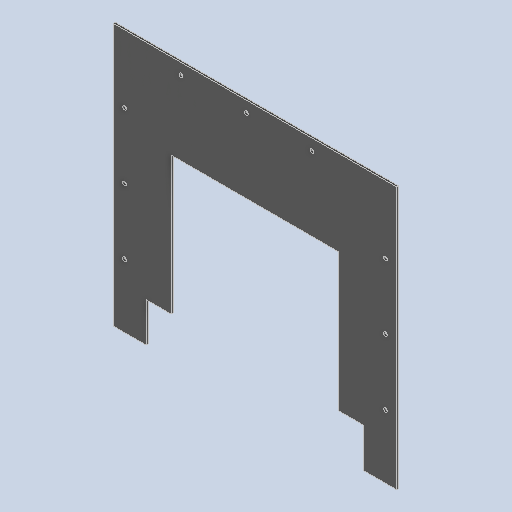
# Autodesk Inventor part: HCMUTE-CDT23-KXL_A03
Saved by Autodesk Inventor 2023 (Build 270158000, 158)
## iProperties
Created: 2023-11-20
Part Number: HCMUTE-CDT23-KXL_A03
Material: PMMA Plastic
Document SubType Name: Modeling
Designer: havie
Density: 1.188 g/cm^3
Appearance: Dark Gray
Author: havie
Autodesk Inventor part; units mm, degrees
ref_plane "YZ Plane" through (0, 0, 0) normal (1, 0, 0) x (0, 1, 0)
ref_plane "XZ Plane" through (0, 0, 0) normal (0, 1, 0) x (-1, 0, 0)
ref_plane "XY Plane" through (0, 0, 0) normal (0, 0, 1) x (1, 0, 0)
sketch "Sketch1" plane through (0, 0, 0) normal (1, 0, 0) x (0, 1, 0)
  line L0 (-216, 200) -> (216, 200)
  line L1 (216, 200) -> (216, -200)
  line L2 (216, -200) -> (-216, -200)
  line L3 (-216, -200) -> (-216, 200)
  line L4 (-216, 200) -> (216, -200) construction
  line L5 (216, 200) -> (-216, -200) construction
  point P0 (0, 0)
  dimension "d0" = 400
  dimension "d1" = 432
  constraints: 12 end point, 2 midpoint, 2 parallel, 1 horizontal, 1 perpendicular
  measures "d0" distance of L0.end L1.end
  measures "d1" distance of L1.end L2.end
extrude "Extrusion1" add sketch "Sketch1" along normal mid plane 3
sketch "Sketch2" plane through (1.5, 0, 0) normal (1, 0, 0) x (0, 0, -1)
  line L0 (200, 216) -> (-200, 216) projected
  line L1 (-200, -216) -> (200, -216) projected
  line L2 (200, -216) -> (200, 216) projected
  line L3 (200, 166) -> (140, 166)
  line L4 (140, 166) -> (140, 128)
  line L5 (140, 128) -> (-70, 128)
  line L6 (-70, 128) -> (-70, -128)
  line L7 (-70, -128) -> (140, -128)
  line L8 (140, -128) -> (140, -166)
  line L9 (140, -166) -> (200, -166)
  point P0 (0, 0)
  dimension "d6" = 50
  dimension "d7" = 50
  dimension "d8" = 60
  dimension "d9" = 38
  dimension "d10" = 270
  constraints: 14 end point, 5 perpendicular, 2 equal length, 2 point on line, 1 horizontal, 1 vertical
  measures "d6" distance between parallel lines of L0 L3
  measures "d7" distance between parallel lines of L1 L9
  measures "d8" distance of L3.start L3.end
  measures "d9" distance of L3.end L4.end
  measures "d10" distance between parallel lines of L2 L6
extrude "Extrusion2" cut sketch "Sketch2" against normal blind 3
sketch "Sketch3" plane through (-1.5, 0, 0) normal (-1, 0, 0) x (0, 0, 1)
  circle A0 centre (97, -199) radius 3
  circle A1 centre (-3, -199) radius 3
  circle A2 centre (-103, -199) radius 3
  line L0 (-200, -216) -> (200, -216) projected
  line L1 (200, -216) -> (200, 216) projected
  point P0 (0, 0)
  dimension "d15" = 6
  dimension "d16" = 6
  dimension "d17" = 6
  dimension "d18" = 17
  dimension "d19" = 103
  dimension "d20" = 100
  dimension "d21" = 100
  constraints: 3 centre point, 2 horizontal alignment
  measures "d15" diameter of A2
  measures "d16" diameter of A1
  measures "d17" diameter of A0
  measures "d18" distance from line of L0 A0.centre
  measures "d19" distance from line of L1 A0.centre
  measures "d20" distance of A1.centre A0.centre
  measures "d21" distance of A2.centre A1.centre
extrude "Extrusion3" cut sketch "Sketch3" against normal blind 3
mirror "Mirror1" about plane through (0, 0, 0) normal (0, 1, 0) of "Extrusion3"
sketch "Sketch4" plane through (-1.5, 0, 0) normal (-1, 0, 0) x (0, 0, 1)
  circle A0 centre (183, 87) radius 2.5 projected
  circle A1 centre (183, -13) radius 2.5 projected
  circle A2 centre (183, -113) radius 2.5 projected
  point P0 (0, 0)
  constraints: 3 coincident
hole "Hole1" at (-1.5, 87, 183) at (-1.5, -13, 183) at (-1.5, -113, 183) direction (1, 0, 0) diameter 6 depth 14.2 tip angle 118
equation "\"d6\" = d7"
body "Solid1"
